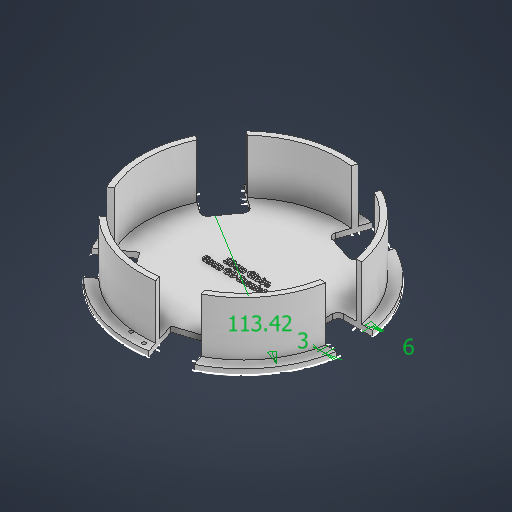
# Autodesk Inventor part: 122mm-CoilForm-6mmCoil
Saved by Autodesk Inventor 2026.1 (Build 301233020, 233B)
## iProperties
Created: 2025-05-18
Part Number: 122mm-CoilForm-6mmCoil
Material: Generic
Document SubType Name: Modeling
Designer: user
Density: 1 g/cm^3
Appearance: Default
Author: user
## iProperties of the stored document 122mm-CoilForm_3DPrint.ipt
Created: 2025-05-18
Part Number: 122mm-CoilForm_3DPrint
Material: Generic
Document SubType Name: Modeling
Designer: user
Density: 1 g/cm^3
Appearance: Default
Author: user
Autodesk Inventor part; units mm, degrees
ref_plane "YZ Plane" through (0, 0, 0) normal (1, 0, 0) x (0, 1, 0)
ref_plane "XZ Plane" through (0, 0, 0) normal (0, 1, 0) x (-1, 0, 0)
ref_plane "XY Plane" through (0, 0, 0) normal (0, 0, 1) x (1, 0, 0)
sketch "Sketch1" plane through (0, 0, 0) normal (0, 1, 0) x (-1, 0, 0)
  circle A0 centre (0, 0) radius 56.71
  circle A1 centre (0, 0) radius 53.71
  circle A2 centre (0, 0) radius 62.71
  dimension "d0" = 113.42
  dimension "d1" = 3
  dimension "d2" = 6
  constraints: 3 centre point, 1 coincident
  measures "d0" diameter of A0
  measures "d1" radial gap between concentric circles of A0 A1
  measures "d2" radial gap between concentric circles of A0 A2
extrude "Extrusion1" add sketch "Sketch1" along normal blind 33 contours A0
extrude "Extrusion2" add sketch "Sketch1" along normal blind 3 contours A2
sketch "Sketch2" plane through (0, 3, 0) normal (0, 1, 0) x (1, 0, 0)
  circle A0 centre (-4.5, -57.5343) radius 1
  circle A1 centre (0, 0) radius 56.71 projected
  circle A2 centre (0, 0) radius 58.71 construction
  circle A3 centre (4.5, -59.5402) radius 1
  dimension "d7" = 2
  dimension "d8" = 4.5
  dimension "d9" = 4.5
  constraints: 3 centre point, 3 tangent, 1 coincident, 1 equal radius
  measures "d7" diameter of A0
  measures "d8" horizontal distance of A0.centre point (0, 0)
  measures "d9" horizontal distance of A3.centre point (0, 0)
extrude "Extrusion3" cut sketch "Sketch2" against normal up to surface (3 mm away) contours A0 | A3
extrude "Extrusion4" add sketch "Sketch1" along normal blind 3 contours A1
sketch "Sketch3" plane through (0, 0, 0) normal (0, -1, 0) x (1, 0, 0)
  line L0 (62.71, -10) -> (42.71, -10)
  line L1 (42.71, -10) -> (42.71, 10)
  line L2 (42.71, 10) -> (62.71, 10)
  line L3 (62.71, 10) -> (62.71, -10)
  circle A0 centre (0, 0) radius 62.71 projected
  point P0 (62.71, 0)
  point P1 (5.4987, 96.2431)
  point P2 (3.5009, 96.3364)
  dimension "d14" = 20
  dimension "d15" = 20
  constraints: 8 end point, 2 parallel, 1 horizontal, 1 horizontal alignment, 1 midpoint, 1 perpendicular, 1 vertical, 1 other
  measures "d14" distance of L2.end L0.start
  measures "d15" distance of L0.start L0.end
extrude "Extrusion5" cut sketch "Sketch3" against normal up to surface (33 mm away) contours L0 A0 L3 | L0 L1 L2 A0 | A0 L2 L3 picked at (49.3767, 0)
pattern_circular "Circular Pattern1" count 5 over 360 about axis through (0, -10, 0) along (0, 1, 0) of "Extrusion5"
fillet "Fillet1" radius 3 6 edges at (42.71, 1.5, 10) (42.71, 1.5, -10) (-40.431, 1.5, -17.0141) (-28.6753, 1.5, -33.1945) (22.7087, 1.5, -37.5295) (3.6876, 1.5, -43.7098)
sketch "Sketch4" plane through (0, 3, 0) normal (0, 1, 0) x (1, 0, 0)
  line L0 (-24.9823, 4.4833) -> (24.5408, 4.4833) construction
  line L1 (24.5408, 4.4833) -> (24.5408, -3.7832) construction
  line L2 (24.5408, -3.7832) -> (-24.9823, -3.7832) construction
  line L3 (-24.9823, -3.7832) -> (-24.9823, 4.4833) construction
  line L4 (-10.2502, 1.2994) -> (-12.2633, 1.2994)
  line L5 (-12.2633, 1.2994) -> (-12.2633, 1.8305)
  line L6 (-12.2633, 1.8305) -> (-11.6211, 1.8305)
  line L7 (-11.6211, 1.8305) -> (-11.6211, 3.4434)
  line L8 (-11.6211, 3.4434) -> (-12.2633, 3.4434)
  line L9 (-12.2633, 3.4434) -> (-12.2633, 3.9399)
  spline S0 degree 2 poles (-12.2633, 3.9399) (-12.1225, 3.9399) (-11.8434, 3.9769) (-11.7594, 4.0165) knots 0 0 0 1 2 2 2
  spline S1 degree 2 poles (-11.7594, 4.0165) (-11.6631, 4.0659) (-11.5544, 4.2314) (-11.5445, 4.3549) knots 0 0 0 1 2 2 2
  line L10 (-11.5445, 4.3549) -> (-10.8776, 4.3549)
  line L11 (-10.8776, 4.3549) -> (-10.8776, 1.8305)
  line L12 (-10.8776, 1.8305) -> (-10.2502, 1.8305)
  line L13 (-10.2502, 1.8305) -> (-10.2502, 1.2994)
  spline S2 degree 2 poles (-7.5209, 2.2232) (-7.5209, 1.9985) (-7.6864, 1.6304) (-7.8469, 1.502) knots 0 0 0 1 2 2 2
  spline S3 degree 2 poles (-7.8469, 1.502) (-8.0075, 1.3735) (-8.4447, 1.2352) (-8.7583, 1.2352) knots 0 0 0 1 2 2 2
  spline S4 degree 2 poles (-8.7583, 1.2352) (-9.114, 1.2352) (-9.6229, 1.3538) (-9.7834, 1.4279) knots 0 0 0 1 2 2 2
  line L14 (-9.7834, 1.4279) -> (-9.7834, 2.0898)
  line L15 (-9.7834, 2.0898) -> (-9.7093, 2.0898)
  spline S5 degree 2 poles (-9.7093, 2.0898) (-9.5413, 1.9836) (-9.0893, 1.8256) (-8.9016, 1.8256) knots 0 0 0 1 2 2 2
  spline S6 degree 2 poles (-8.9016, 1.8256) (-8.7905, 1.8256) (-8.5311, 1.8651) (-8.4422, 1.9293) knots 0 0 0 1 2 2 2
  spline S7 degree 2 poles (-8.4422, 1.9293) (-8.373, 1.9812) (-8.289, 2.1318) (-8.289, 2.2677) knots 0 0 0 1 2 2 2
  spline S8 degree 2 poles (-8.289, 2.2677) (-8.289, 2.4035) (-8.4076, 2.5493) (-8.5064, 2.5839) knots 0 0 0 1 2 2 2
  spline S9 degree 2 poles (-8.5064, 2.5839) (-8.6052, 2.6184) (-8.8794, 2.6258) (-8.9856, 2.6258) knots 0 0 0 1 2 2 2
  line L16 (-8.9856, 2.6258) -> (-9.1165, 2.6258)
  line L17 (-9.1165, 2.6258) -> (-9.1165, 3.1618)
  line L18 (-9.1165, 3.1618) -> (-8.9955, 3.1618)
  spline S10 degree 2 poles (-8.9955, 3.1618) (-8.8571, 3.1618) (-8.6225, 3.1865) (-8.541, 3.2236) knots 0 0 0 1 2 2 2
  spline S11 degree 2 poles (-8.541, 3.2236) (-8.4595, 3.2631) (-8.3681, 3.4014) (-8.3681, 3.52) knots 0 0 0 1 2 2 2
  spline S12 degree 2 poles (-8.3681, 3.52) (-8.3681, 3.6138) (-8.4545, 3.7299) (-8.5163, 3.762) knots 0 0 0 1 2 2 2
  spline S13 degree 2 poles (-8.5163, 3.762) (-8.5904, 3.7991) (-8.788, 3.8238) (-8.8571, 3.8238) knots 0 0 0 1 2 2 2
  spline S14 degree 2 poles (-8.8571, 3.8238) (-8.9683, 3.8238) (-9.2029, 3.7719) (-9.3116, 3.7299) knots 0 0 0 1 2 2 2
  spline S15 degree 2 poles (-9.3116, 3.7299) (-9.3981, 3.6978) (-9.5858, 3.5941) (-9.6303, 3.5669) knots 0 0 0 1 2 2 2
  line L19 (-9.6303, 3.5669) -> (-9.6945, 3.5669)
  line L20 (-9.6945, 3.5669) -> (-9.6945, 4.219)
  spline S16 degree 2 poles (-9.6945, 4.219) (-9.5364, 4.2857) (-9.0029, 4.4117) (-8.7238, 4.4117) knots 0 0 0 1 2 2 2
  spline S17 degree 2 poles (-8.7238, 4.4117) (-8.4521, 4.4117) (-8.0519, 4.3178) (-7.9111, 4.2264) knots 0 0 0 1 2 2 2
  spline S18 degree 2 poles (-7.9111, 4.2264) (-7.7555, 4.1301) (-7.5999, 3.8337) (-7.5999, 3.6484) knots 0 0 0 1 2 2 2
  spline S19 degree 2 poles (-7.5999, 3.6484) (-7.5999, 3.3866) (-7.9012, 2.9963) (-8.1483, 2.9395) knots 0 0 0 1 2 2 2
  line L21 (-8.1483, 2.9395) -> (-8.1483, 2.9099)
  spline S20 degree 2 poles (-8.1483, 2.9099) (-8.0396, 2.8951) (-7.8321, 2.816) (-7.7333, 2.7271) knots 0 0 0 1 2 2 2
  spline S21 degree 2 poles (-7.7333, 2.7271) (-7.6419, 2.6481) (-7.5209, 2.3961) (-7.5209, 2.2232) knots 0 0 0 1 2 2 2
  spline S22 degree 2 poles (-5.9228, 1.2377) (-6.2068, 1.2377) (-6.6786, 1.381) (-6.854, 1.5292) knots 0 0 0 1 2 2 2
  spline S23 degree 2 poles (-6.854, 1.5292) (-7.0244, 1.6798) (-7.2171, 2.1318) (-7.2171, 2.4381) knots 0 0 0 1 2 2 2
  spline S24 degree 2 poles (-7.2171, 2.4381) (-7.2171, 2.7691) (-7.0096, 3.231) (-6.8293, 3.3792) knots 0 0 0 1 2 2 2
  spline S25 degree 2 poles (-6.8293, 3.3792) (-6.6588, 3.5225) (-6.1945, 3.6608) (-5.9425, 3.6608) knots 0 0 0 1 2 2 2
  spline S26 degree 2 poles (-5.9425, 3.6608) (-5.7523, 3.6608) (-5.372, 3.5719) (-5.1793, 3.4755) knots 0 0 0 1 2 2 2
  line L22 (-5.1793, 3.4755) -> (-5.1793, 2.863)
  line L23 (-5.1793, 2.863) -> (-5.2707, 2.863)
  spline S27 degree 2 poles (-5.2707, 2.863) (-5.3151, 2.905) (-5.4386, 3.0038) (-5.5127, 3.0433) knots 0 0 0 1 2 2 2
  spline S28 degree 2 poles (-5.5127, 3.0433) (-5.5918, 3.0877) (-5.7869, 3.147) (-5.9079, 3.147) knots 0 0 0 1 2 2 2
  spline S29 degree 2 poles (-5.9079, 3.147) (-6.1821, 3.147) (-6.4835, 2.7642) (-6.4835, 2.4381) knots 0 0 0 1 2 2 2
  spline S30 degree 2 poles (-6.4835, 2.4381) (-6.4835, 2.0923) (-6.1624, 1.7515) (-5.8956, 1.7515) knots 0 0 0 1 2 2 2
  spline S31 degree 2 poles (-5.8956, 1.7515) (-5.7597, 1.7515) (-5.5572, 1.8132) (-5.4831, 1.8577) knots 0 0 0 1 2 2 2
  spline S32 degree 2 poles (-5.4831, 1.8577) (-5.4115, 1.8997) (-5.3077, 1.9935) (-5.2707, 2.0306) knots 0 0 0 1 2 2 2
  line L24 (-5.2707, 2.0306) -> (-5.1793, 2.0306)
  line L25 (-5.1793, 2.0306) -> (-5.1793, 1.4155)
  spline S33 degree 2 poles (-5.1793, 1.4155) (-5.241, 1.3884) (-5.4016, 1.3192) (-5.4856, 1.297) knots 0 0 0 1 2 2 2
  spline S34 degree 2 poles (-5.4856, 1.297) (-5.5893, 1.2673) (-5.7721, 1.2377) (-5.9228, 1.2377) knots 0 0 0 1 2 2 2
  line L26 (-2.0942, 1.2994) -> (-2.0942, 2.448)
  spline S35 degree 2 poles (-2.0942, 2.448) (-2.0942, 2.6184) (-2.1066, 2.8506) (-2.1362, 2.9247) knots 0 0 0 1 2 2 2
  spline S36 degree 2 poles (-2.1362, 2.9247) (-2.1683, 2.9988) (-2.2968, 3.0655) (-2.4129, 3.0655) knots 0 0 0 1 2 2 2
  spline S37 degree 2 poles (-2.4129, 3.0655) (-2.4944, 3.0655) (-2.6525, 2.9939) (-2.7463, 2.9272) knots 0 0 0 1 2 2 2
  line L27 (-2.7463, 2.9272) -> (-2.7463, 1.2994)
  line L28 (-2.7463, 1.2994) -> (-3.4676, 1.2994)
  line L29 (-3.4676, 1.2994) -> (-3.4676, 2.448)
  spline S38 degree 2 poles (-3.4676, 2.448) (-3.4676, 2.616) (-3.4824, 2.8506) (-3.512, 2.9247) knots 0 0 0 1 2 2 2
  spline S39 degree 2 poles (-3.512, 2.9247) (-3.5441, 2.9988) (-3.6726, 3.0655) (-3.7887, 3.0655) knots 0 0 0 1 2 2 2
  spline S40 degree 2 poles (-3.7887, 3.0655) (-3.8751, 3.0655) (-4.0456, 2.984) (-4.1246, 2.9272) knots 0 0 0 1 2 2 2
  line L30 (-4.1246, 2.9272) -> (-4.1246, 1.2994)
  line L31 (-4.1246, 1.2994) -> (-4.8409, 1.2994)
  line L32 (-4.8409, 1.2994) -> (-4.8409, 3.599)
  line L33 (-4.8409, 3.599) -> (-4.1246, 3.599)
  line L34 (-4.1246, 3.599) -> (-4.1246, 3.3446)
  spline S41 degree 2 poles (-4.1246, 3.3446) (-3.9492, 3.4928) (-3.6355, 3.6608) (-3.4404, 3.6608) knots 0 0 0 1 2 2 2
  spline S42 degree 2 poles (-3.4404, 3.6608) (-3.2304, 3.6608) (-2.9093, 3.4607) (-2.8254, 3.2606) knots 0 0 0 1 2 2 2
  spline S43 degree 2 poles (-2.8254, 3.2606) (-2.6204, 3.4533) (-2.2548, 3.6608) (-2.0671, 3.6608) knots 0 0 0 1 2 2 2
  spline S44 degree 2 poles (-2.0671, 3.6608) (-1.9065, 3.6608) (-1.6521, 3.5595) (-1.5657, 3.4558) knots 0 0 0 1 2 2 2
  spline S45 degree 2 poles (-1.5657, 3.4558) (-1.4693, 3.3446) (-1.373, 3.0408) (-1.373, 2.7963) knots 0 0 0 1 2 2 2
  line L35 (-1.373, 2.7963) -> (-1.373, 1.2994)
  line L36 (-1.373, 1.2994) -> (-2.0942, 1.2994)
  spline S46 degree 2 poles (2.9718, 1.4723) (2.7717, 1.3908) (2.132, 1.2352) (1.8207, 1.2352) knots 0 0 0 1 2 2 2
  spline S47 degree 2 poles (1.8207, 1.2352) (1.102, 1.2352) (0.2498, 2.0651) (0.2498, 2.8259) knots 0 0 0 1 2 2 2
  spline S48 degree 2 poles (0.2498, 2.8259) (0.2498, 3.5422) (1.102, 4.4067) (1.843, 4.4067) knots 0 0 0 1 2 2 2
  spline S49 degree 2 poles (1.843, 4.4067) (2.2258, 4.4067) (2.705, 4.261) (2.9594, 4.1375) knots 0 0 0 1 2 2 2
  line L37 (2.9594, 4.1375) -> (2.9594, 3.4212)
  line L38 (2.9594, 3.4212) -> (2.8903, 3.4212)
  spline S50 degree 2 poles (2.8903, 3.4212) (2.8359, 3.4632) (2.6284, 3.6237) (2.5296, 3.6781) knots 0 0 0 1 2 2 2
  spline S51 degree 2 poles (2.5296, 3.6781) (2.416, 3.7448) (2.1147, 3.8386) (1.9467, 3.8386) knots 0 0 0 1 2 2 2
  spline S52 degree 2 poles (1.9467, 3.8386) (1.7516, 3.8386) (1.428, 3.7151) (1.302, 3.5891) knots 0 0 0 1 2 2 2
  spline S53 degree 2 poles (1.302, 3.5891) (1.181, 3.4656) (1.0402, 3.0877) (1.0402, 2.8383) knots 0 0 0 1 2 2 2
  spline S54 degree 2 poles (1.0402, 2.8383) (1.0402, 2.3047) (1.5762, 1.7959) (2.0381, 1.7959) knots 0 0 0 1 2 2 2
  spline S55 degree 2 poles (2.0381, 1.7959) (2.0801, 1.7959) (2.1888, 1.8009) (2.2308, 1.8033) knots 0 0 0 1 2 2 2
  line L39 (2.2308, 1.8033) -> (2.2308, 2.4035)
  line L40 (2.2308, 2.4035) -> (1.6404, 2.4035)
  line L41 (1.6404, 2.4035) -> (1.6404, 2.9741)
  line L42 (1.6404, 2.9741) -> (2.9718, 2.9741)
  line L43 (2.9718, 2.9741) -> (2.9718, 1.4723)
  line L44 (4.2241, 1.2994) -> (3.5078, 1.2994)
  line L45 (3.5078, 1.2994) -> (3.5078, 4.4833)
  line L46 (3.5078, 4.4833) -> (4.2241, 4.4833)
  line L47 (4.2241, 4.4833) -> (4.2241, 1.2994)
  spline S56 degree 2 poles (6.9781, 2.448) (6.9781, 1.8799) (6.3582, 1.2278) (5.7925, 1.2278) knots 0 0 0 1 2 2 2
  spline S57 degree 2 poles (5.7925, 1.2278) (5.2294, 1.2278) (4.6044, 1.8799) (4.6044, 2.448) knots 0 0 0 1 2 2 2
  spline S58 degree 2 poles (4.6044, 2.448) (4.6044, 3.021) (5.2294, 3.6707) (5.7925, 3.6707) knots 0 0 0 1 2 2 2
  spline S59 degree 2 poles (5.7925, 3.6707) (6.3557, 3.6707) (6.9781, 3.0186) (6.9781, 2.448) knots 0 0 0 1 2 2 2
  spline S60 degree 2 poles (6.2445, 2.4431) (6.2445, 2.6481) (6.1778, 2.9222) (6.1186, 3.0038) knots 0 0 0 1 2 2 2
  spline S61 degree 2 poles (6.1186, 3.0038) (6.0543, 3.0902) (5.8938, 3.1569) (5.7925, 3.1569) knots 0 0 0 1 2 2 2
  spline S62 degree 2 poles (5.7925, 3.1569) (5.6937, 3.1569) (5.5381, 3.0976) (5.4739, 3.0136) knots 0 0 0 1 2 2 2
  spline S63 degree 2 poles (5.4739, 3.0136) (5.4121, 2.9346) (5.338, 2.6555) (5.338, 2.4431) knots 0 0 0 1 2 2 2
  spline S64 degree 2 poles (5.338, 2.4431) (5.338, 2.2331) (5.4072, 1.9738) (5.464, 1.8947) knots 0 0 0 1 2 2 2
  spline S65 degree 2 poles (5.464, 1.8947) (5.5208, 1.8157) (5.6937, 1.7416) (5.7975, 1.7416) knots 0 0 0 1 2 2 2
  spline S66 degree 2 poles (5.7975, 1.7416) (5.8839, 1.7416) (6.0618, 1.8157) (6.1161, 1.8898) knots 0 0 0 1 2 2 2
  spline S67 degree 2 poles (6.1161, 1.8898) (6.1778, 1.9762) (6.2445, 2.2257) (6.2445, 2.4431) knots 0 0 0 1 2 2 2
  spline S68 degree 2 poles (9.6112, 2.4801) (9.6112, 1.9318) (9.0554, 1.255) (8.6429, 1.255) knots 0 0 0 1 2 2 2
  spline S69 degree 2 poles (8.6429, 1.255) (8.4725, 1.255) (8.2181, 1.3316) (8.0748, 1.4131) knots 0 0 0 1 2 2 2
  line L48 (8.0748, 1.4131) -> (8.0452, 1.2994)
  line L49 (8.0452, 1.2994) -> (7.3585, 1.2994)
  line L50 (7.3585, 1.2994) -> (7.3585, 4.4833)
  line L51 (7.3585, 4.4833) -> (8.0748, 4.4833)
  line L52 (8.0748, 4.4833) -> (8.0748, 3.357)
  spline S70 degree 2 poles (8.0748, 3.357) (8.2329, 3.4928) (8.5589, 3.6608) (8.7738, 3.6608) knots 0 0 0 1 2 2 2
  spline S71 degree 2 poles (8.7738, 3.6608) (9.1764, 3.6608) (9.6112, 3.0359) (9.6112, 2.4801) knots 0 0 0 1 2 2 2
  spline S72 degree 2 poles (8.8776, 2.4653) (8.8776, 2.8086) (8.6701, 3.1026) (8.4527, 3.1026) knots 0 0 0 1 2 2 2
  spline S73 degree 2 poles (8.4527, 3.1026) (8.3564, 3.1026) (8.1662, 3.0408) (8.0748, 2.9791) knots 0 0 0 1 2 2 2
  line L53 (8.0748, 2.9791) -> (8.0748, 1.828)
  spline S74 degree 2 poles (8.0748, 1.828) (8.1464, 1.7984) (8.2922, 1.7786) (8.3638, 1.7786) knots 0 0 0 1 2 2 2
  spline S75 degree 2 poles (8.3638, 1.7786) (8.6232, 1.7786) (8.8776, 2.122) (8.8776, 2.4653) knots 0 0 0 1 2 2 2
  spline S76 degree 2 poles (11.1846, 1.2377) (10.5325, 1.2377) (9.8384, 1.8601) (9.8384, 2.4357) knots 0 0 0 1 2 2 2
  spline S77 degree 2 poles (9.8384, 2.4357) (9.8384, 2.9988) (10.4856, 3.6707) (11.0685, 3.6707) knots 0 0 0 1 2 2 2
  spline S78 degree 2 poles (11.0685, 3.6707) (11.5946, 3.6707) (12.1281, 3.1001) (12.1281, 2.5715) knots 0 0 0 1 2 2 2
  line L54 (12.1281, 2.5715) -> (12.1281, 2.3122)
  line L55 (12.1281, 2.3122) -> (10.5547, 2.3122)
  spline S79 degree 2 poles (10.5547, 2.3122) (10.5646, 2.1516) (10.6807, 1.9392) (10.7745, 1.875) knots 0 0 0 1 2 2 2
  spline S80 degree 2 poles (10.7745, 1.875) (10.8659, 1.8107) (11.1129, 1.7564) (11.2587, 1.7564) knots 0 0 0 1 2 2 2
  spline S81 degree 2 poles (11.2587, 1.7564) (11.3822, 1.7564) (11.6242, 1.8107) (11.7255, 1.8577) knots 0 0 0 1 2 2 2
  spline S82 degree 2 poles (11.7255, 1.8577) (11.8144, 1.8947) (11.9626, 1.9861) (12.0096, 2.0207) knots 0 0 0 1 2 2 2
  line L56 (12.0096, 2.0207) -> (12.0861, 2.0207)
  line L57 (12.0861, 2.0207) -> (12.0861, 1.4279)
  spline S83 degree 2 poles (12.0861, 1.4279) (11.9972, 1.3933) (11.8539, 1.334) (11.7255, 1.3044) knots 0 0 0 1 2 2 2
  spline S84 degree 2 poles (11.7255, 1.3044) (11.6094, 1.2723) (11.3624, 1.2377) (11.1846, 1.2377) knots 0 0 0 1 2 2 2
  spline S85 degree 2 poles (11.4217, 2.7444) (11.4167, 2.9716) (11.2167, 3.2112) (11.0117, 3.2112) knots 0 0 0 1 2 2 2
  spline S86 degree 2 poles (11.0117, 3.2112) (10.8017, 3.2112) (10.5646, 2.9593) (10.5522, 2.7444) knots 0 0 0 1 2 2 2
  line L58 (10.5522, 2.7444) -> (11.4217, 2.7444)
  spline S87 degree 2 poles (-17.1823, -2.6816) (-17.1823, -3.1633) (-17.7924, -3.7832) (-18.326, -3.7832) knots 0 0 0 1 2 2 2
  spline S88 degree 2 poles (-18.326, -3.7832) (-18.5927, -3.7832) (-19.0101, -3.6301) (-19.1559, -3.4794) knots 0 0 0 1 2 2 2
  spline S89 degree 2 poles (-19.1559, -3.4794) (-19.3288, -3.304) (-19.514, -2.7483) (-19.514, -2.3605) knots 0 0 0 1 2 2 2
  spline S90 degree 2 poles (-19.514, -2.3605) (-19.514, -1.9604) (-19.3411, -1.3379) (-19.146, -1.0983) knots 0 0 0 1 2 2 2
  spline S91 degree 2 poles (-19.146, -1.0983) (-18.9607, -0.8711) (-18.3581, -0.6142) (-17.9456, -0.6142) knots 0 0 0 1 2 2 2
  spline S92 degree 2 poles (-17.9456, -0.6142) (-17.7949, -0.6142) (-17.4936, -0.6537) (-17.4392, -0.6661) knots 0 0 0 1 2 2 2
  line L59 (-17.4392, -0.6661) -> (-17.4392, -1.2638)
  line L60 (-17.4392, -1.2638) -> (-17.4936, -1.2638)
  spline S93 degree 2 poles (-17.4936, -1.2638) (-17.5479, -1.2366) (-17.7949, -1.17) (-17.953, -1.17) knots 0 0 0 1 2 2 2
  spline S94 degree 2 poles (-17.953, -1.17) (-18.3111, -1.17) (-18.7014, -1.5479) (-18.7483, -1.8986) knots 0 0 0 1 2 2 2
  spline S95 degree 2 poles (-18.7483, -1.8986) (-18.5977, -1.8023) (-18.2889, -1.6887) (-18.0938, -1.6887) knots 0 0 0 1 2 2 2
  spline S96 degree 2 poles (-18.0938, -1.6887) (-17.9283, -1.6887) (-17.6393, -1.7776) (-17.5281, -1.8616) knots 0 0 0 1 2 2 2
  spline S97 degree 2 poles (-17.5281, -1.8616) (-17.3701, -1.9826) (-17.1823, -2.3753) (-17.1823, -2.6816) knots 0 0 0 1 2 2 2
  spline S98 degree 2 poles (-18.074, -3.141) (-18.0147, -3.0669) (-17.9505, -2.894) (-17.9505, -2.7187) knots 0 0 0 1 2 2 2
  spline S99 degree 2 poles (-17.9505, -2.7187) (-17.9505, -2.5705) (-18.0246, -2.3778) (-18.0913, -2.321) knots 0 0 0 1 2 2 2
  spline S100 degree 2 poles (-18.0913, -2.321) (-18.1605, -2.2617) (-18.3309, -2.2197) (-18.4272, -2.2197) knots 0 0 0 1 2 2 2
  spline S101 degree 2 poles (-18.4272, -2.2197) (-18.5087, -2.2197) (-18.6767, -2.2617) (-18.7508, -2.2913) knots 0 0 0 1 2 2 2
  spline S102 degree 2 poles (-18.7508, -2.2913) (-18.7508, -2.3111) (-18.7557, -2.405) (-18.7557, -2.4766) knots 0 0 0 1 2 2 2
  spline S103 degree 2 poles (-18.7557, -2.4766) (-18.7557, -2.7409) (-18.6643, -3.0595) (-18.5927, -3.141) knots 0 0 0 1 2 2 2
  spline S104 degree 2 poles (-18.5927, -3.141) (-18.5408, -3.2077) (-18.4025, -3.2645) (-18.3284, -3.2645) knots 0 0 0 1 2 2 2
  spline S105 degree 2 poles (-18.3284, -3.2645) (-18.2667, -3.2645) (-18.1234, -3.2028) (-18.074, -3.141) knots 0 0 0 1 2 2 2
  line L61 (-14.0257, -3.719) -> (-14.0257, -2.5705)
  spline S106 degree 2 poles (-14.0257, -2.5705) (-14.0257, -2.4) (-14.038, -2.1678) (-14.0676, -2.0937) knots 0 0 0 1 2 2 2
  spline S107 degree 2 poles (-14.0676, -2.0937) (-14.0998, -2.0196) (-14.2282, -1.9529) (-14.3443, -1.9529) knots 0 0 0 1 2 2 2
  spline S108 degree 2 poles (-14.3443, -1.9529) (-14.4258, -1.9529) (-14.5839, -2.0246) (-14.6777, -2.0913) knots 0 0 0 1 2 2 2
  line L62 (-14.6777, -2.0913) -> (-14.6777, -3.719)
  line L63 (-14.6777, -3.719) -> (-15.399, -3.719)
  line L64 (-15.399, -3.719) -> (-15.399, -2.5705)
  spline S109 degree 2 poles (-15.399, -2.5705) (-15.399, -2.4025) (-15.4138, -2.1678) (-15.4434, -2.0937) knots 0 0 0 1 2 2 2
  spline S110 degree 2 poles (-15.4434, -2.0937) (-15.4756, -2.0196) (-15.604, -1.9529) (-15.7201, -1.9529) knots 0 0 0 1 2 2 2
  spline S111 degree 2 poles (-15.7201, -1.9529) (-15.8065, -1.9529) (-15.977, -2.0345) (-16.056, -2.0913) knots 0 0 0 1 2 2 2
  line L65 (-16.056, -2.0913) -> (-16.056, -3.719)
  line L66 (-16.056, -3.719) -> (-16.7723, -3.719)
  line L67 (-16.7723, -3.719) -> (-16.7723, -1.4194)
  line L68 (-16.7723, -1.4194) -> (-16.056, -1.4194)
  line L69 (-16.056, -1.4194) -> (-16.056, -1.6738)
  spline S112 degree 2 poles (-16.056, -1.6738) (-15.8806, -1.5256) (-15.5669, -1.3577) (-15.3718, -1.3577) knots 0 0 0 1 2 2 2
  spline S113 degree 2 poles (-15.3718, -1.3577) (-15.1619, -1.3577) (-14.8408, -1.5577) (-14.7568, -1.7578) knots 0 0 0 1 2 2 2
  spline S114 degree 2 poles (-14.7568, -1.7578) (-14.5518, -1.5652) (-14.1862, -1.3577) (-13.9985, -1.3577) knots 0 0 0 1 2 2 2
  spline S115 degree 2 poles (-13.9985, -1.3577) (-13.8379, -1.3577) (-13.5835, -1.4589) (-13.4971, -1.5627) knots 0 0 0 1 2 2 2
  spline S116 degree 2 poles (-13.4971, -1.5627) (-13.4007, -1.6738) (-13.3044, -1.9776) (-13.3044, -2.2222) knots 0 0 0 1 2 2 2
  line L70 (-13.3044, -2.2222) -> (-13.3044, -3.719)
  line L71 (-13.3044, -3.719) -> (-14.0257, -3.719)
  line L72 (-10.0292, -3.719) -> (-10.0292, -2.5705)
  spline S117 degree 2 poles (-10.0292, -2.5705) (-10.0292, -2.4) (-10.0415, -2.1678) (-10.0712, -2.0937) knots 0 0 0 1 2 2 2
  spline S118 degree 2 poles (-10.0712, -2.0937) (-10.1033, -2.0196) (-10.2317, -1.9529) (-10.3478, -1.9529) knots 0 0 0 1 2 2 2
  spline S119 degree 2 poles (-10.3478, -1.9529) (-10.4293, -1.9529) (-10.5874, -2.0246) (-10.6813, -2.0913) knots 0 0 0 1 2 2 2
  line L73 (-10.6813, -2.0913) -> (-10.6813, -3.719)
  line L74 (-10.6813, -3.719) -> (-11.4025, -3.719)
  line L75 (-11.4025, -3.719) -> (-11.4025, -2.5705)
  spline S120 degree 2 poles (-11.4025, -2.5705) (-11.4025, -2.4025) (-11.4173, -2.1678) (-11.447, -2.0937) knots 0 0 0 1 2 2 2
  spline S121 degree 2 poles (-11.447, -2.0937) (-11.4791, -2.0196) (-11.6075, -1.9529) (-11.7236, -1.9529) knots 0 0 0 1 2 2 2
  spline S122 degree 2 poles (-11.7236, -1.9529) (-11.81, -1.9529) (-11.9805, -2.0345) (-12.0595, -2.0913) knots 0 0 0 1 2 2 2
  line L76 (-12.0595, -2.0913) -> (-12.0595, -3.719)
  line L77 (-12.0595, -3.719) -> (-12.7758, -3.719)
  line L78 (-12.7758, -3.719) -> (-12.7758, -1.4194)
  line L79 (-12.7758, -1.4194) -> (-12.0595, -1.4194)
  line L80 (-12.0595, -1.4194) -> (-12.0595, -1.6738)
  spline S123 degree 2 poles (-12.0595, -1.6738) (-11.8842, -1.5256) (-11.5705, -1.3577) (-11.3753, -1.3577) knots 0 0 0 1 2 2 2
  spline S124 degree 2 poles (-11.3753, -1.3577) (-11.1654, -1.3577) (-10.8443, -1.5577) (-10.7603, -1.7578) knots 0 0 0 1 2 2 2
  spline S125 degree 2 poles (-10.7603, -1.7578) (-10.5553, -1.5652) (-10.1897, -1.3577) (-10.002, -1.3577) knots 0 0 0 1 2 2 2
  spline S126 degree 2 poles (-10.002, -1.3577) (-9.8414, -1.3577) (-9.587, -1.4589) (-9.5006, -1.5627) knots 0 0 0 1 2 2 2
  spline S127 degree 2 poles (-9.5006, -1.5627) (-9.4043, -1.6738) (-9.3079, -1.9776) (-9.3079, -2.2222) knots 0 0 0 1 2 2 2
  line L81 (-9.3079, -2.2222) -> (-9.3079, -3.719)
  line L82 (-9.3079, -3.719) -> (-10.0292, -3.719)
  spline S128 degree 2 poles (-4.7335, -2.195) (-4.7335, -2.936) (-5.5239, -3.7832) (-6.2105, -3.7832) knots 0 0 0 1 2 2 2
  spline S129 degree 2 poles (-6.2105, -3.7832) (-6.8997, -3.7832) (-7.6851, -2.9261) (-7.6851, -2.195) knots 0 0 0 1 2 2 2
  spline S130 degree 2 poles (-7.6851, -2.195) (-7.6851, -1.4614) (-6.8997, -0.6068) (-6.2105, -0.6068) knots 0 0 0 1 2 2 2
  spline S131 degree 2 poles (-6.2105, -0.6068) (-5.5239, -0.6068) (-4.7335, -1.4565) (-4.7335, -2.195) knots 0 0 0 1 2 2 2
  spline S132 degree 2 poles (-5.5239, -2.195) (-5.5239, -1.9208) (-5.635, -1.538) (-5.7313, -1.417) knots 0 0 0 1 2 2 2
  spline S133 degree 2 poles (-5.7313, -1.417) (-5.8277, -1.291) (-6.0747, -1.1823) (-6.2081, -1.1823) knots 0 0 0 1 2 2 2
  spline S134 degree 2 poles (-6.2081, -1.1823) (-6.3488, -1.1823) (-6.5786, -1.2836) (-6.6848, -1.412) knots 0 0 0 1 2 2 2
  spline S135 degree 2 poles (-6.6848, -1.412) (-6.7786, -1.5306) (-6.8947, -1.9233) (-6.8947, -2.195) knots 0 0 0 1 2 2 2
  spline S136 degree 2 poles (-6.8947, -2.195) (-6.8947, -2.4766) (-6.7836, -2.8471) (-6.6872, -2.9731) knots 0 0 0 1 2 2 2
  spline S137 degree 2 poles (-6.6872, -2.9731) (-6.5909, -3.099) (-6.3414, -3.2077) (-6.2081, -3.2077) knots 0 0 0 1 2 2 2
  spline S138 degree 2 poles (-6.2081, -3.2077) (-6.0722, -3.2077) (-5.8203, -3.0916) (-5.7289, -2.9681) knots 0 0 0 1 2 2 2
  spline S139 degree 2 poles (-5.7289, -2.9681) (-5.6301, -2.8347) (-5.5239, -2.4815) (-5.5239, -2.195) knots 0 0 0 1 2 2 2
  spline S140 degree 2 poles (-1.5595, -2.1975) (-1.5595, -2.6248) (-1.9325, -3.2966) (-2.2165, -3.4769) knots 0 0 0 1 2 2 2
  spline S141 degree 2 poles (-2.2165, -3.4769) (-2.4536, -3.6301) (-3.0119, -3.719) (-3.3255, -3.719) knots 0 0 0 1 2 2 2
  line L83 (-3.3255, -3.719) -> (-4.279, -3.719)
  line L84 (-4.279, -3.719) -> (-4.279, -0.671)
  line L85 (-4.279, -0.671) -> (-3.3354, -0.671)
  spline S142 degree 2 poles (-3.3354, -0.671) (-3.0143, -0.671) (-2.4536, -0.7525) (-2.2066, -0.9106) knots 0 0 0 1 2 2 2
  spline S143 degree 2 poles (-2.2066, -0.9106) (-1.9078, -1.1033) (-1.5595, -1.7553) (-1.5595, -2.1975) knots 0 0 0 1 2 2 2
  spline S144 degree 2 poles (-2.3449, -2.1925) (-2.3449, -1.8912) (-2.5524, -1.4614) (-2.7649, -1.3404) knots 0 0 0 1 2 2 2
  spline S145 degree 2 poles (-2.7649, -1.3404) (-2.9205, -1.2564) (-3.2613, -1.2391) (-3.4984, -1.2391) knots 0 0 0 1 2 2 2
  line L86 (-3.4984, -1.2391) -> (-3.5133, -1.2391)
  line L87 (-3.5133, -1.2391) -> (-3.5133, -3.1484)
  line L88 (-3.5133, -3.1484) -> (-3.4984, -3.1484)
  spline S146 degree 2 poles (-3.4984, -3.1484) (-3.2416, -3.1484) (-2.8884, -3.1311) (-2.7278, -3.0299) knots 0 0 0 1 2 2 2
  spline S147 degree 2 poles (-2.7278, -3.0299) (-2.5401, -2.9113) (-2.3449, -2.4939) (-2.3449, -2.1925) knots 0 0 0 1 2 2 2
  line L89 (1.6392, -3.719) -> (-0.0009, -3.719)
  line L90 (-0.0009, -3.719) -> (-0.0009, -3.188)
  line L91 (-0.0009, -3.188) -> (0.4363, -3.188)
  line L92 (0.4363, -3.188) -> (0.4363, -1.2021)
  line L93 (0.4363, -1.2021) -> (-0.0009, -1.2021)
  line L94 (-0.0009, -1.2021) -> (-0.0009, -0.671)
  line L95 (-0.0009, -0.671) -> (1.6392, -0.671)
  line L96 (1.6392, -0.671) -> (1.6392, -1.2021)
  line L97 (1.6392, -1.2021) -> (1.202, -1.2021)
  line L98 (1.202, -1.2021) -> (1.202, -3.188)
  line L99 (1.202, -3.188) -> (1.6392, -3.188)
  line L100 (1.6392, -3.188) -> (1.6392, -3.719)
  line L101 (4.2574, -3.719) -> (3.5362, -3.719)
  line L102 (3.5362, -3.719) -> (3.5362, -2.5803)
  spline S148 degree 2 poles (3.5362, -2.5803) (3.5362, -2.4395) (3.5139, -2.1629) (3.4843, -2.0987) knots 0 0 0 1 2 2 2
  spline S149 degree 2 poles (3.4843, -2.0987) (3.4472, -2.0196) (3.3089, -1.9529) (3.1904, -1.9529) knots 0 0 0 1 2 2 2
  spline S150 degree 2 poles (3.1904, -1.9529) (3.1039, -1.9529) (2.9236, -2.0196) (2.8223, -2.0913) knots 0 0 0 1 2 2 2
  line L103 (2.8223, -2.0913) -> (2.8223, -3.719)
  line L104 (2.8223, -3.719) -> (2.106, -3.719)
  line L105 (2.106, -3.719) -> (2.106, -1.4194)
  line L106 (2.106, -1.4194) -> (2.8223, -1.4194)
  line L107 (2.8223, -1.4194) -> (2.8223, -1.6738)
  spline S151 degree 2 poles (2.8223, -1.6738) (2.9977, -1.5256) (3.3311, -1.3577) (3.5337, -1.3577) knots 0 0 0 1 2 2 2
  spline S152 degree 2 poles (3.5337, -1.3577) (3.8844, -1.3577) (4.2574, -1.8023) (4.2574, -2.2222) knots 0 0 0 1 2 2 2
  line L108 (4.2574, -2.2222) -> (4.2574, -3.719)
  spline S153 degree 2 poles (5.4875, -3.7808) (5.2355, -3.7808) (4.7835, -3.6696) (4.6353, -3.5955) knots 0 0 0 1 2 2 2
  line L109 (4.6353, -3.5955) -> (4.6353, -2.9904)
  line L110 (4.6353, -2.9904) -> (4.6946, -2.9904)
  spline S154 degree 2 poles (4.6946, -2.9904) (4.7465, -3.0299) (4.8774, -3.1237) (4.9935, -3.1756) knots 0 0 0 1 2 2 2
  spline S155 degree 2 poles (4.9935, -3.1756) (5.0947, -3.2225) (5.3442, -3.2892) (5.4924, -3.2892) knots 0 0 0 1 2 2 2
  spline S156 degree 2 poles (5.4924, -3.2892) (5.6431, -3.2892) (5.8753, -3.1954) (5.8753, -3.0941) knots 0 0 0 1 2 2 2
  spline S157 degree 2 poles (5.8753, -3.0941) (5.8753, -3.0151) (5.7691, -2.9311) (5.6159, -2.8965) knots 0 0 0 1 2 2 2
  spline S158 degree 2 poles (5.6159, -2.8965) (5.5344, -2.8743) (5.2849, -2.8273) (5.1886, -2.7977) knots 0 0 0 1 2 2 2
  spline S159 degree 2 poles (5.1886, -2.7977) (4.9169, -2.7137) (4.6452, -2.3852) (4.6452, -2.116) knots 0 0 0 1 2 2 2
  spline S160 degree 2 poles (4.6452, -2.116) (4.6452, -1.9628) (4.786, -1.6911) (4.9243, -1.5849) knots 0 0 0 1 2 2 2
  spline S161 degree 2 poles (4.9243, -1.5849) (5.0602, -1.4812) (5.4628, -1.3577) (5.7172, -1.3577) knots 0 0 0 1 2 2 2
  spline S162 degree 2 poles (5.7172, -1.3577) (5.9592, -1.3577) (6.3643, -1.454) (6.5027, -1.5207) knots 0 0 0 1 2 2 2
  line L111 (6.5027, -1.5207) -> (6.5027, -2.1036)
  line L112 (6.5027, -2.1036) -> (6.4458, -2.1036)
  spline S163 degree 2 poles (6.4458, -2.1036) (6.4088, -2.074) (6.2482, -1.9776) (6.1741, -1.9431) knots 0 0 0 1 2 2 2
  spline S164 degree 2 poles (6.1741, -1.9431) (6.0827, -1.9035) (5.8604, -1.8492) (5.7444, -1.8492) knots 0 0 0 1 2 2 2
  spline S165 degree 2 poles (5.7444, -1.8492) (5.5887, -1.8492) (5.3739, -1.9554) (5.3739, -2.0419) knots 0 0 0 1 2 2 2
  spline S166 degree 2 poles (5.3739, -2.0419) (5.3739, -2.1209) (5.4801, -2.2098) (5.6579, -2.2543) knots 0 0 0 1 2 2 2
  spline S167 degree 2 poles (5.6579, -2.2543) (5.7493, -2.2765) (5.9889, -2.3185) (6.1, -2.3556) knots 0 0 0 1 2 2 2
  spline S168 degree 2 poles (6.1, -2.3556) (6.347, -2.4346) (6.6039, -2.7434) (6.6039, -3.0002) knots 0 0 0 1 2 2 2
  spline S169 degree 2 poles (6.6039, -3.0002) (6.6039, -3.1608) (6.4533, -3.4547) (6.3125, -3.5535) knots 0 0 0 1 2 2 2
  spline S170 degree 2 poles (6.3125, -3.5535) (6.1667, -3.6622) (5.7666, -3.7808) (5.4875, -3.7808) knots 0 0 0 1 2 2 2
  line L113 (9.0789, -3.719) -> (8.3626, -3.719)
  line L114 (8.3626, -3.719) -> (8.3626, -3.4646)
  spline S171 degree 2 poles (8.3626, -3.4646) (8.1773, -3.6202) (7.8661, -3.7832) (7.6512, -3.7832) knots 0 0 0 1 2 2 2
  spline S172 degree 2 poles (7.6512, -3.7832) (7.3103, -3.7832) (6.9275, -3.351) (6.9275, -2.9163) knots 0 0 0 1 2 2 2
  line L115 (6.9275, -2.9163) -> (6.9275, -1.4194)
  line L116 (6.9275, -1.4194) -> (7.6487, -1.4194)
  line L117 (7.6487, -1.4194) -> (7.6487, -2.5606)
  spline S173 degree 2 poles (7.6487, -2.5606) (7.6487, -2.7384) (7.666, -2.9657) (7.7006, -3.0422) knots 0 0 0 1 2 2 2
  spline S174 degree 2 poles (7.7006, -3.0422) (7.7352, -3.1139) (7.871, -3.188) (7.9945, -3.188) knots 0 0 0 1 2 2 2
  spline S175 degree 2 poles (7.9945, -3.188) (8.0686, -3.188) (8.2761, -3.1139) (8.3626, -3.0496) knots 0 0 0 1 2 2 2
  line L118 (8.3626, -3.0496) -> (8.3626, -1.4194)
  line L119 (8.3626, -1.4194) -> (9.0789, -1.4194)
  line L120 (9.0789, -1.4194) -> (9.0789, -3.719)
  line L121 (10.3435, -3.719) -> (9.6272, -3.719)
  line L122 (9.6272, -3.719) -> (9.6272, -0.5352)
  line L123 (9.6272, -0.5352) -> (10.3435, -0.5352)
  line L124 (10.3435, -0.5352) -> (10.3435, -3.719)
  spline S176 degree 2 poles (12.159, -3.4745) (12.0849, -3.5362) (11.9688, -3.635) (11.87, -3.6844) knots 0 0 0 1 2 2 2
  spline S177 degree 2 poles (11.87, -3.6844) (11.7737, -3.7314) (11.5909, -3.7808) (11.4279, -3.7808) knots 0 0 0 1 2 2 2
  spline S178 degree 2 poles (11.4279, -3.7808) (11.1216, -3.7808) (10.719, -3.3707) (10.719, -3.0595) knots 0 0 0 1 2 2 2
  spline S179 degree 2 poles (10.719, -3.0595) (10.719, -2.8051) (10.924, -2.4889) (11.1166, -2.3975) knots 0 0 0 1 2 2 2
  spline S180 degree 2 poles (11.1166, -2.3975) (11.3118, -2.3037) (11.8527, -2.2296) (12.1639, -2.2098) knots 0 0 0 1 2 2 2
  line L125 (12.1639, -2.2098) -> (12.1639, -2.1975)
  spline S181 degree 2 poles (12.1639, -2.1975) (12.1639, -2.0073) (11.8823, -1.8616) (11.6008, -1.8616) knots 0 0 0 1 2 2 2
  spline S182 degree 2 poles (11.6008, -1.8616) (11.4748, -1.8616) (11.1339, -1.9529) (10.9734, -2.0246) knots 0 0 0 1 2 2 2
  line L126 (10.9734, -2.0246) -> (10.9116, -2.0246)
  line L127 (10.9116, -2.0246) -> (10.9116, -1.4688)
  spline S183 degree 2 poles (10.9116, -1.4688) (11.0178, -1.4392) (11.4921, -1.3552) (11.7341, -1.3552) knots 0 0 0 1 2 2 2
  spline S184 degree 2 poles (11.7341, -1.3552) (12.3269, -1.3552) (12.8704, -1.7504) (12.8704, -2.1555) knots 0 0 0 1 2 2 2
  line L128 (12.8704, -2.1555) -> (12.8704, -3.719)
  line L129 (12.8704, -3.719) -> (12.159, -3.719)
  line L130 (12.159, -3.719) -> (12.159, -3.4745)
  line L131 (12.159, -3.1188) -> (12.159, -2.6421)
  spline S185 degree 2 poles (12.159, -2.6421) (11.9762, -2.6594) (11.7514, -2.6865) (11.6428, -2.7261) knots 0 0 0 1 2 2 2
  spline S186 degree 2 poles (11.6428, -2.7261) (11.5464, -2.7582) (11.4427, -2.8916) (11.4427, -3.0002) knots 0 0 0 1 2 2 2
  spline S187 degree 2 poles (11.4427, -3.0002) (11.4427, -3.1608) (11.6181, -3.2818) (11.7885, -3.2818) knots 0 0 0 1 2 2 2
  spline S188 degree 2 poles (11.7885, -3.2818) (11.8823, -3.2818) (12.0799, -3.1954) (12.159, -3.1188) knots 0 0 0 1 2 2 2
  spline S189 degree 2 poles (14.2807, -3.7635) (13.8435, -3.7635) (13.4434, -3.4028) (13.4434, -2.9928) knots 0 0 0 1 2 2 2
  line L132 (13.4434, -2.9928) -> (13.4434, -1.9184)
  line L133 (13.4434, -1.9184) -> (13.1692, -1.9184)
  line L134 (13.1692, -1.9184) -> (13.1692, -1.4194)
  line L135 (13.1692, -1.4194) -> (13.4434, -1.4194)
  line L136 (13.4434, -1.4194) -> (13.4434, -0.7624)
  line L137 (13.4434, -0.7624) -> (14.1597, -0.7624)
  line L138 (14.1597, -0.7624) -> (14.1597, -1.4194)
  line L139 (14.1597, -1.4194) -> (14.8513, -1.4194)
  line L140 (14.8513, -1.4194) -> (14.8513, -1.9184)
  line L141 (14.8513, -1.9184) -> (14.1597, -1.9184)
  line L142 (14.1597, -1.9184) -> (14.1597, -2.7359)
  spline S190 degree 2 poles (14.1597, -2.7359) (14.1597, -2.857) (14.1646, -3.0373) (14.1943, -3.1089) knots 0 0 0 1 2 2 2
  spline S191 degree 2 poles (14.1943, -3.1089) (14.2239, -3.1805) (14.3697, -3.2645) (14.508, -3.2645) knots 0 0 0 1 2 2 2
  spline S192 degree 2 poles (14.508, -3.2645) (14.5673, -3.2645) (14.7525, -3.2151) (14.7896, -3.1954) knots 0 0 0 1 2 2 2
  line L143 (14.7896, -3.1954) -> (14.8513, -3.1954)
  line L144 (14.8513, -3.1954) -> (14.8513, -3.6992)
  spline S193 degree 2 poles (14.8513, -3.6992) (14.7352, -3.7289) (14.4734, -3.7635) (14.2807, -3.7635) knots 0 0 0 1 2 2 2
  spline S194 degree 2 poles (17.3485, -2.5705) (17.3485, -3.1386) (16.7285, -3.7906) (16.1629, -3.7906) knots 0 0 0 1 2 2 2
  spline S195 degree 2 poles (16.1629, -3.7906) (15.5997, -3.7906) (14.9748, -3.1386) (14.9748, -2.5705) knots 0 0 0 1 2 2 2
  spline S196 degree 2 poles (14.9748, -2.5705) (14.9748, -1.9974) (15.5997, -1.3478) (16.1629, -1.3478) knots 0 0 0 1 2 2 2
  spline S197 degree 2 poles (16.1629, -1.3478) (16.726, -1.3478) (17.3485, -1.9999) (17.3485, -2.5705) knots 0 0 0 1 2 2 2
  spline S198 degree 2 poles (16.6149, -2.5754) (16.6149, -2.3704) (16.5482, -2.0962) (16.4889, -2.0147) knots 0 0 0 1 2 2 2
  spline S199 degree 2 poles (16.4889, -2.0147) (16.4247, -1.9282) (16.2642, -1.8616) (16.1629, -1.8616) knots 0 0 0 1 2 2 2
  spline S200 degree 2 poles (16.1629, -1.8616) (16.0641, -1.8616) (15.9085, -1.9208) (15.8443, -2.0048) knots 0 0 0 1 2 2 2
  spline S201 degree 2 poles (15.8443, -2.0048) (15.7825, -2.0839) (15.7084, -2.363) (15.7084, -2.5754) knots 0 0 0 1 2 2 2
  spline S202 degree 2 poles (15.7084, -2.5754) (15.7084, -2.7853) (15.7776, -3.0447) (15.8344, -3.1237) knots 0 0 0 1 2 2 2
  spline S203 degree 2 poles (15.8344, -3.1237) (15.8912, -3.2028) (16.0641, -3.2769) (16.1678, -3.2769) knots 0 0 0 1 2 2 2
  spline S204 degree 2 poles (16.1678, -3.2769) (16.2543, -3.2769) (16.4321, -3.2028) (16.4865, -3.1287) knots 0 0 0 1 2 2 2
  spline S205 degree 2 poles (16.4865, -3.1287) (16.5482, -3.0422) (16.6149, -2.7928) (16.6149, -2.5754) knots 0 0 0 1 2 2 2
  line L145 (19.2726, -2.0987) -> (19.2134, -2.0987)
  spline S206 degree 2 poles (19.2134, -2.0987) (19.1714, -2.0839) (19.0158, -2.069) (18.9219, -2.069) knots 0 0 0 1 2 2 2
  spline S207 degree 2 poles (18.9219, -2.069) (18.8107, -2.069) (18.5613, -2.1357) (18.4452, -2.1802) knots 0 0 0 1 2 2 2
  line L146 (18.4452, -2.1802) -> (18.4452, -3.719)
  line L147 (18.4452, -3.719) -> (17.7289, -3.719)
  line L148 (17.7289, -3.719) -> (17.7289, -1.4194)
  line L149 (17.7289, -1.4194) -> (18.4452, -1.4194)
  line L150 (18.4452, -1.4194) -> (18.4452, -1.7504)
  spline S208 degree 2 poles (18.4452, -1.7504) (18.4946, -1.7059) (18.6675, -1.5676) (18.7391, -1.5256) knots 0 0 0 1 2 2 2
  spline S209 degree 2 poles (18.7391, -1.5256) (18.8182, -1.4787) (19.0256, -1.412) (19.117, -1.412) knots 0 0 0 1 2 2 2
  spline S210 degree 2 poles (19.117, -1.412) (19.1516, -1.412) (19.2381, -1.417) (19.2726, -1.4194) knots 0 0 0 1 2 2 2
  line L151 (19.2726, -1.4194) -> (19.2726, -2.0987)
  point P0 (0, 0)
  constraints: 2 other
extrude "Extrusion6" add sketch "Sketch4" along normal blind 1
body "Solid1"
